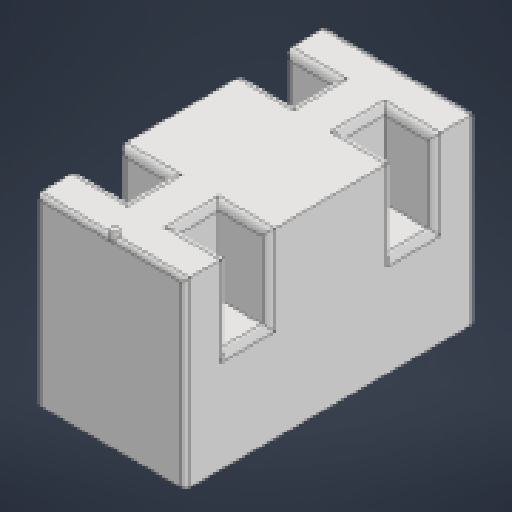
# Autodesk Inventor part: SACMI DPA C-RAIL BOTTOM SUPPORT
Saved by Autodesk Inventor 2025 (Build 290162000, 162)
## iProperties
Created: 2024-05-18
Part Number: SACMI DPA C-RAIL BOTTOM SUPPORT
Material: Generic
Document SubType Name: Modeling
Designer: zulet
Density: 1 g/cm^3
Appearance: Default
Author: zulet
Autodesk Inventor part; units mm, degrees
ref_plane "YZ Plane" through (0, 0, 0) normal (1, 0, 0) x (0, 1, 0)
ref_plane "XZ Plane" through (0, 0, 0) normal (0, 1, 0) x (-1, 0, 0)
ref_plane "XY Plane" through (0, 0, 0) normal (0, 0, 1) x (1, 0, 0)
sketch "Sketch1" plane through (0, 0, 0) normal (0, 1, 0) x (-1, 0, 0)
  line L0 (0, 0) -> (90, 0) construction
  line L1 (90, 0) -> (90, 175)
  line L2 (90, 175) -> (0, 175)
  line L3 (0, 175) -> (0, 0) construction
  line L4 (90, 125) -> (0, 125)
  line L5 (0, 125) -> (0, 75) construction
  line L6 (0, 75) -> (90, 75)
  line L7 (90, 75) -> (90, 125)
  line L8 (30, 125) -> (30, 75)
  line L9 (27.5, 75) -> (62.5, 75) construction
  line L10 (62.5, 75) -> (62.5, 125) construction
  line L11 (62.5, 125) -> (27.5, 125) construction
  line L12 (27.5, 125) -> (27.5, 75) construction
  line L13 (27.5, 75) -> (62.5, 125) construction
  line L14 (62.5, 75) -> (27.5, 125) construction
  line L15 (90, 0) -> (90, -175)
  line L16 (90, -175) -> (0, -175)
  line L17 (90, -125) -> (0, -125)
  line L18 (0, -75) -> (90, -75)
  line L19 (90, -75) -> (90, -125)
  line L20 (30, -125) -> (30, -75)
  line L21 (27.5, -75) -> (62.5, -75) construction
  line L22 (62.5, -75) -> (62.5, -125) construction
  line L23 (62.5, -125) -> (27.5, -125) construction
  line L24 (27.5, -125) -> (27.5, -75) construction
  line L25 (27.5, -75) -> (62.5, -125) construction
  line L26 (62.5, -75) -> (27.5, -125) construction
  line L27 (-90, 0) -> (-90, 175)
  line L28 (-90, 175) -> (0, 175)
  line L29 (-90, 125) -> (0, 125)
  line L30 (0, 75) -> (-90, 75)
  line L31 (-90, 75) -> (-90, 125)
  line L32 (-30, 125) -> (-30, 75)
  line L33 (-27.5, 75) -> (-62.5, 75) construction
  line L34 (-62.5, 75) -> (-62.5, 125) construction
  line L35 (-62.5, 125) -> (-27.5, 125) construction
  line L36 (-27.5, 125) -> (-27.5, 75) construction
  line L37 (-27.5, 75) -> (-62.5, 125) construction
  line L38 (-62.5, 75) -> (-27.5, 125) construction
  line L39 (-90, 0) -> (-90, -175)
  line L40 (-90, -175) -> (0, -175)
  line L41 (-90, -125) -> (0, -125)
  line L42 (0, -75) -> (-90, -75)
  line L43 (-90, -75) -> (-90, -125)
  line L44 (-30, -125) -> (-30, -75)
  line L45 (-27.5, -75) -> (-62.5, -75) construction
  line L46 (-62.5, -75) -> (-62.5, -125) construction
  line L47 (-62.5, -125) -> (-27.5, -125) construction
  line L48 (-27.5, -125) -> (-27.5, -75) construction
  line L49 (-27.5, -75) -> (-62.5, -125) construction
  line L50 (-62.5, -75) -> (-27.5, -125) construction
  line L51 (45, 100) -> (90, 100) construction
  point P0 (45, -100)
  point P1 (-45, 100)
  point P2 (-45, -100)
  point P3 (45, -100)
  point P4 (-45, 100)
  dimension "d0" = 200
  dimension "d1" = 35
  dimension "d2" = 50
  dimension "d3" = 90
  dimension "d4" = 180
  dimension "d5" = 50
  dimension "d6" = 50
  dimension "d7" = 60
  constraints: 104 end point, 46 symmetric about line, 16 coincident, 13 point on line, 6 parallel, 5 midpoint, 4 horizontal, 4 perpendicular
  measures "d0" distance of point (45, -100) L51.start
  measures "d1" distance of L10.end L11.end
  measures "d2" distance of L9.end L10.end
  measures "d3" distance of point (-45, 100) L51.start
  measures "d4" distance between parallel lines of L27 L1
  measures "d5" distance between parallel lines of L6 L4
  measures "d6" distance between parallel lines of L2 L11
  measures "d7" distance between parallel lines of L32 L8
extrude "Extrusion1" add sketch "Sketch1" along normal blind 220 contours L15 L18 L42 L39 L27 L30 L6 L1 | L4 L29 L27 L28 L2 L1 | L6 L30 L32 L29 L4 L8 | L15 L16 L40 L39 L41 L17 | L20 L17 L41 L44 L42 L18
extrude "Extrusion2" add sketch "Sketch1" along normal blind 120 contours L6 L8 L4 L1 | L15 L17 L20 L18 | L30 L27 L29 L32 | L44 L41 L39 L42
hole "Hole1" at (-62.5, 0, 125) at (-27.5, 0, 125) at (-27.5, 0, 75) at (-62.5, 0, 75) at (-62.5, 0, -75) at (-27.5, 0, -75) at (-27.5, 0, -125) at (-62.5, 0, -125) at (62.5, 0, 75) at (27.5, 0, 75) at (27.5, 0, 125) at (62.5, 0, 125) at (62.5, 0, -125) at (27.5, 0, -125) at (27.5, 0, -75) at (62.5, 0, -75) direction (0, 1, 0) diameter 8 depth 15
fillet "Fillet1" radius 5 6 edges at (0, 220, -175) (-90, 110, -175) (90, 110, -175) (-90, 110, 175) (0, 220, 175) (90, 110, 175)
fillet "Fillet2" radius 8 24 edges at (-60, 220, -125) (-90, 170, -125) (-60, 220, -75) (-90, 170, -75) (-90, 120, -100) (-30, 220, -100) (-60, 220, 75) (-30, 220, 100) (-60, 220, 125) (-90, 170, 75) (-90, 120, 100) (-90, 170, 125) (60, 220, -75) (30, 220, -100) (60, 220, -125) (60, 220, 75) (30, 220, 100) (60, 220, 125) (90, 170, 75) (90, 170, 125) (90, 120, 100) (90, 170, -75) (90, 120, -100) (90, 170, -125)
sketch "Sketch2" plane through (0, 220, 0) normal (0, 1, 0) x (1, 0, 0)
  line L0 (90, -170) -> (-90, -170) projected
  circle A0 centre (0, -170) radius 5
  point P0 (0, 0)
  dimension "d21" = 10
  constraints: 1 centre point, 1 midpoint
  measures "d21" diameter of A0
extrude "Extrusion3" add sketch "Sketch2" along normal mid plane 10
body "Solid1"
